Autodesk Inventor part; units mm, degrees
(part 2 of 3)
sketch "Sketch1" plane through (0, 0, 0) normal (0, 1, 0) x (-1, 0, 0)
  circle A0 centre (0, 0) radius 7.7717
  line L0 (3.8714, 3.1643) -> (5.8376, 5.1305)
  line L1 (3.1643, 3.8714) -> (5.1305, 5.8376)
  line L2 (-3.1643, -3.8714) -> (-5.1305, -5.8376)
  line L3 (-3.8714, -3.1643) -> (-5.8376, -5.1305)
  line L4 (3.1643, -3.8714) -> (5.1305, -5.8376)
  line L5 (5.8376, -5.1305) -> (3.8714, -3.1643)
  line L6 (-3.8714, 3.1643) -> (-5.8376, 5.1305)
  line L7 (-3.1643, 3.8714) -> (-5.1305, 5.8376)
  line L8 (0, 0) -> (0, -3.4995) construction
  line L9 (0, 0) -> (1.6685, -1.6685) construction
  circle A1 centre (0, 0) radius 5
  line L10 (0, 0) -> (2.6888, 2.6888) construction
  line L11 (4.7918, 7.3512) -> (4.9104, 7.3218)
  line L12 (4.9104, 7.3218) -> (4.97, 7.3308)
  line L13 (4.97, 7.3308) -> (5.0192, 7.3467)
  line L14 (5.0192, 7.3467) -> (5.0629, 7.3663)
  line L15 (5.0629, 7.3663) -> (5.1027, 7.3884)
  line L16 (5.1027, 7.3884) -> (5.1747, 7.4379)
  line L17 (5.1747, 7.4379) -> (5.2391, 7.4925)
  line L18 (5.2391, 7.4925) -> (5.2982, 7.5509)
  line L19 (5.2982, 7.5509) -> (5.3528, 7.6123)
  line L20 (5.3528, 7.6123) -> (5.456, 7.7394)
  line L21 (5.456, 7.7394) -> (5.5742, 7.8558)
  line L22 (5.5742, 7.8558) -> (5.7038, 7.964)
  line L23 (5.7038, 7.964) -> (5.8421, 8.0657)
  line L24 (5.8421, 8.0657) -> (5.9879, 8.1615)
  line L25 (5.9879, 8.1615) -> (6.1405, 8.2518)
  line L26 (6.1405, 8.2518) -> (6.2994, 8.3368)
  line L27 (6.2994, 8.3368) -> (6.4641, 8.4166)
  line L28 (6.4641, 8.4166) -> (6.6342, 8.4914)
  line L29 (6.6342, 8.4914) -> (6.8096, 8.5612)
  line L30 (6.8096, 8.5612) -> (6.9898, 8.6259)
  line L31 (6.9898, 8.6259) -> (7.1281, 8.6711)
  line L32 (7.1281, 8.6711) -> (7.4493, 8.3968)
  line L33 (7.4493, 8.3968) -> (7.4262, 8.2531)
  line L34 (7.4262, 8.2531) -> (7.3905, 8.065)
  line L35 (7.3905, 8.065) -> (7.3491, 7.8809)
  line L36 (7.3491, 7.8809) -> (7.3018, 7.7011)
  line L37 (7.3018, 7.7011) -> (7.2487, 7.526)
  line L38 (7.2487, 7.526) -> (7.1896, 7.3558)
  line L39 (7.1896, 7.3558) -> (7.1243, 7.1909)
  line L40 (7.1243, 7.1909) -> (7.0525, 7.0319)
  line L41 (7.0525, 7.0319) -> (6.9737, 6.8794)
  line L42 (6.9737, 6.8794) -> (6.8871, 6.7345)
  line L43 (6.8871, 6.7345) -> (6.7906, 6.5995)
  line L44 (6.7906, 6.5995) -> (6.6812, 6.4777)
  line L45 (6.6812, 6.4777) -> (6.6291, 6.4142)
  line L46 (6.6291, 6.4142) -> (6.5807, 6.3467)
  line L47 (6.5807, 6.3467) -> (6.5369, 6.2745)
  line L48 (6.5369, 6.2745) -> (6.4992, 6.1957)
  line L49 (6.4992, 6.1957) -> (6.4836, 6.1529)
  line L50 (6.4836, 6.1529) -> (6.4711, 6.1067)
  line L51 (6.4711, 6.1067) -> (6.4631, 6.0556)
  line L52 (6.4631, 6.0556) -> (6.4635, 5.9953)
  line L53 (6.4635, 5.9953) -> (6.5111, 5.8828)
  line L54 (6.5111, 5.8828) -> (6.829, 5.5107)
  line L55 (6.829, 5.5107) -> (6.9326, 5.446)
  line L56 (6.9326, 5.446) -> (6.9921, 5.4362)
  line L57 (6.9921, 5.4362) -> (7.0439, 5.4361)
  line L58 (7.0439, 5.4361) -> (7.0914, 5.4413)
  line L59 (7.0914, 5.4413) -> (7.1361, 5.45)
  line L60 (7.1361, 5.45) -> (7.2198, 5.4748)
  line L61 (7.2198, 5.4748) -> (7.298, 5.5068)
  line L62 (7.298, 5.5068) -> (7.3722, 5.5441)
  line L63 (7.3722, 5.5441) -> (7.4432, 5.5856)
  line L64 (7.4432, 5.5856) -> (7.5805, 5.6746)
  line L65 (7.5805, 5.6746) -> (7.729, 5.7488)
  line L66 (7.729, 5.7488) -> (7.8856, 5.8117)
  line L67 (7.8856, 5.8117) -> (8.0486, 5.8656)
  line L68 (8.0486, 5.8656) -> (8.2169, 5.9116)
  line L69 (8.2169, 5.9116) -> (8.3899, 5.9504)
  line L70 (8.3899, 5.9504) -> (8.5673, 5.9821)
  line L71 (8.5673, 5.9821) -> (8.7486, 6.0072)
  line L72 (8.7486, 6.0072) -> (8.9335, 6.0257)
  line L73 (8.9335, 6.0257) -> (9.1218, 6.0379)
  line L74 (9.1218, 6.0379) -> (9.3133, 6.0437)
  line L75 (9.3133, 6.0437) -> (9.4588, 6.044)
  line L76 (9.4588, 6.044) -> (9.6794, 5.6839)
  line L77 (9.6794, 5.6839) -> (9.6131, 5.5544)
  line L78 (9.6131, 5.5544) -> (9.521, 5.3864)
  line L79 (9.521, 5.3864) -> (9.4247, 5.2242)
  line L80 (9.4247, 5.2242) -> (9.3242, 5.0678)
  line L81 (9.3242, 5.0678) -> (9.2196, 4.9177)
  line L82 (9.2196, 4.9177) -> (9.1108, 4.7741)
  line L83 (9.1108, 4.7741) -> (8.9977, 4.6375)
  line L84 (8.9977, 4.6375) -> (8.8803, 4.5084)
  line L85 (8.8803, 4.5084) -> (8.7582, 4.3877)
  line L86 (8.7582, 4.3877) -> (8.6311, 4.2767)
  line L87 (8.6311, 4.2767) -> (8.4976, 4.1781)
  line L88 (8.4976, 4.1781) -> (8.3559, 4.0961)
  line L89 (8.3559, 4.0961) -> (8.2867, 4.0517)
  line L90 (8.2867, 4.0517) -> (8.2199, 4.0026)
  line L91 (8.2199, 4.0026) -> (8.1559, 3.9474)
  line L92 (8.1559, 3.9474) -> (8.0957, 3.8841)
  line L93 (8.0957, 3.8841) -> (8.0676, 3.8482)
  line L94 (8.0676, 3.8482) -> (8.0414, 3.8082)
  line L95 (8.0414, 3.8082) -> (8.0181, 3.762)
  line L96 (8.0181, 3.762) -> (7.9998, 3.7046)
  line L97 (7.9998, 3.7046) -> (8.0103, 3.5829)
  line L98 (8.0103, 3.5829) -> (8.1976, 3.1307)
  line L99 (8.1976, 3.1307) -> (8.2762, 3.0372)
  line L100 (8.2762, 3.0372) -> (8.3298, 3.0095)
  line L101 (8.3298, 3.0095) -> (8.3789, 2.9934)
  line L102 (8.3789, 2.9934) -> (8.4258, 2.9836)
  line L103 (8.4258, 2.9836) -> (8.471, 2.9781)
  line L104 (8.471, 2.9781) -> (8.5583, 2.9758)
  line L105 (8.5583, 2.9758) -> (8.6426, 2.9821)
  line L106 (8.6426, 2.9821) -> (8.7246, 2.9946)
  line L107 (8.7246, 2.9946) -> (8.8049, 3.0122)
  line L108 (8.8049, 3.0122) -> (8.9631, 3.0544)
  line L109 (8.9631, 3.0544) -> (9.1272, 3.0791)
  line L110 (9.1272, 3.0791) -> (9.2956, 3.0905)
  line L111 (9.2956, 3.0905) -> (9.4672, 3.0914)
  line L112 (9.4672, 3.0914) -> (9.6415, 3.0832)
  line L113 (9.6415, 3.0832) -> (9.8181, 3.0665)
  line L114 (9.8181, 3.0665) -> (9.9966, 3.0419)
  line L115 (9.9966, 3.0419) -> (10.1767, 3.0097)
  line L116 (10.1767, 3.0097) -> (10.3583, 2.9702)
  line L117 (10.3583, 2.9702) -> (10.5412, 2.9236)
  line L118 (10.5412, 2.9236) -> (10.7251, 2.87)
  line L119 (10.7251, 2.87) -> (10.8635, 2.8253)
  line L120 (10.8635, 2.8253) -> (10.9621, 2.4146)
  line L121 (10.9621, 2.4146) -> (10.859, 2.3119)
  line L122 (10.859, 2.3119) -> (10.7195, 2.1807)
  line L123 (10.7195, 2.1807) -> (10.5778, 2.0561)
  line L124 (10.5778, 2.0561) -> (10.4339, 1.9385)
  line L125 (10.4339, 1.9385) -> (10.288, 1.828)
  line L126 (10.288, 1.828) -> (10.1401, 1.725)
  line L127 (10.1401, 1.725) -> (9.9904, 1.63)
  line L128 (9.9904, 1.63) -> (9.8388, 1.5436)
  line L129 (9.8388, 1.5436) -> (9.6855, 1.4665)
  line L130 (9.6855, 1.4665) -> (9.5302, 1.4002)
  line L131 (9.5302, 1.4002) -> (9.3728, 1.3477)
  line L132 (9.3728, 1.3477) -> (9.2127, 1.3135)
  line L133 (9.2127, 1.3135) -> (9.1332, 1.2927)
  line L134 (9.1332, 1.2927) -> (9.0544, 1.2666)
  line L135 (9.0544, 1.2666) -> (8.9765, 1.2339)
  line L136 (8.9765, 1.2339) -> (8.8997, 1.1923)
  line L137 (8.8997, 1.1923) -> (8.8619, 1.1668)
  line L138 (8.8619, 1.1668) -> (8.8247, 1.1368)
  line L139 (8.8247, 1.1368) -> (8.7882, 1.1002)
  line L140 (8.7882, 1.1002) -> (8.753, 1.0512)
  line L141 (8.753, 1.0512) -> (8.7254, 0.9322)
  line L142 (8.7254, 0.9322) -> (8.7638, 0.4443)
  line L143 (8.7638, 0.4443) -> (8.8097, 0.331)
  line L144 (8.8097, 0.331) -> (8.8521, 0.2881)
  line L145 (8.8521, 0.2881) -> (8.8939, 0.2576)
  line L146 (8.8939, 0.2576) -> (8.9354, 0.2339)
  line L147 (8.9354, 0.2339) -> (8.9767, 0.2146)
  line L148 (8.9767, 0.2146) -> (9.059, 0.1855)
  line L149 (9.059, 0.1855) -> (9.1411, 0.1654)
  line L150 (9.1411, 0.1654) -> (9.223, 0.152)
  line L151 (9.223, 0.152) -> (9.3048, 0.1439)
  line L152 (9.3048, 0.1439) -> (9.4682, 0.1351)
  line L153 (9.4682, 0.1351) -> (9.6319, 0.1079)
  line L154 (9.6319, 0.1079) -> (9.7956, 0.0667)
  line L155 (9.7956, 0.0667) -> (9.9592, 0.0146)
  line L156 (9.9592, 0.0146) -> (10.1224, -0.0471)
  line L157 (10.1224, -0.0471) -> (10.2851, -0.1175)
  line L158 (10.2851, -0.1175) -> (10.4473, -0.1961)
  line L159 (10.4473, -0.1961) -> (10.6087, -0.2824)
  line L160 (10.6087, -0.2824) -> (10.7692, -0.3761)
  line L161 (10.7692, -0.3761) -> (10.9287, -0.4769)
  line L162 (10.9287, -0.4769) -> (11.087, -0.5847)
  line L163 (11.087, -0.5847) -> (11.2049, -0.67)
  line L164 (11.2049, -0.67) -> (11.1718, -1.0911)
  line L165 (11.1718, -1.0911) -> (11.042, -1.1569)
  line L166 (11.042, -1.1569) -> (10.8687, -1.2386)
  line L167 (10.8687, -1.2386) -> (10.6955, -1.3132)
  line L168 (10.6955, -1.3132) -> (10.5223, -1.3807)
  line L169 (10.5223, -1.3807) -> (10.3493, -1.4406)
  line L170 (10.3493, -1.4406) -> (10.1769, -1.4929)
  line L171 (10.1769, -1.4929) -> (10.0051, -1.5369)
  line L172 (10.0051, -1.5369) -> (9.8343, -1.5723)
  line L173 (9.8343, -1.5723) -> (9.6646, -1.5983)
  line L174 (9.6646, -1.5983) -> (9.4965, -1.6134)
  line L175 (9.4965, -1.6134) -> (9.3305, -1.6146)
  line L176 (9.3305, -1.6146) -> (9.1677, -1.5977)
  line L177 (9.1677, -1.5977) -> (9.0856, -1.5929)
  line L178 (9.0856, -1.5929) -> (9.0026, -1.5934)
  line L179 (9.0026, -1.5934) -> (8.9185, -1.6004)
  line L180 (8.9185, -1.6004) -> (8.8326, -1.6162)
  line L181 (8.8326, -1.6162) -> (8.7888, -1.6288)
  line L182 (8.7888, -1.6288) -> (8.744, -1.6458)
  line L183 (8.744, -1.6458) -> (8.698, -1.6694)
  line L184 (8.698, -1.6694) -> (8.6495, -1.7051)
  line L185 (8.6495, -1.7051) -> (8.5864, -1.8098)
  line L186 (8.5864, -1.8098) -> (8.4722, -2.2857)
  line L187 (8.4722, -2.2857) -> (8.4808, -2.4075)
  line L188 (8.4808, -2.4075) -> (8.5079, -2.4614)
  line L189 (8.5079, -2.4614) -> (8.5382, -2.5033)
  line L190 (8.5382, -2.5033) -> (8.5703, -2.5388)
  line L191 (8.5703, -2.5388) -> (8.6037, -2.5698)
  line L192 (8.6037, -2.5698) -> (8.673, -2.6229)
  line L193 (8.673, -2.6229) -> (8.7448, -2.6674)
  line L194 (8.7448, -2.6674) -> (8.8185, -2.7055)
  line L195 (8.8185, -2.7055) -> (8.8938, -2.7385)
  line L196 (8.8938, -2.7385) -> (9.0466, -2.7973)
  line L197 (9.0466, -2.7973) -> (9.1938, -2.8738)
  line L198 (9.1938, -2.8738) -> (9.3368, -2.9636)
  line L199 (9.3368, -2.9636) -> (9.4762, -3.0637)
  line L200 (9.4762, -3.0637) -> (9.6124, -3.1728)
  line L201 (9.6124, -3.1728) -> (9.7454, -3.2901)
  line L202 (9.7454, -3.2901) -> (9.8754, -3.4149)
  line L203 (9.8754, -3.4149) -> (10.0022, -3.5468)
  line L204 (10.0022, -3.5468) -> (10.1259, -3.6855)
  line L205 (10.1259, -3.6855) -> (10.2464, -3.8307)
  line L206 (10.2464, -3.8307) -> (10.3637, -3.9822)
  line L207 (10.3637, -3.9822) -> (10.4494, -4.0997)
  line L208 (10.4494, -4.0997) -> (10.2878, -4.4899)
  line L209 (10.2878, -4.4899) -> (10.1441, -4.5124)
  line L210 (10.1441, -4.5124) -> (9.954, -4.5366)
  line L211 (9.954, -4.5366) -> (9.7662, -4.554)
  line L212 (9.7662, -4.554) -> (9.5806, -4.5647)
  line L213 (9.5806, -4.5647) -> (9.3976, -4.5683)
  line L214 (9.3976, -4.5683) -> (9.2175, -4.5646)
  line L215 (9.2175, -4.5646) -> (9.0405, -4.5535)
  line L216 (9.0405, -4.5535) -> (8.8671, -4.5343)
  line L217 (8.8671, -4.5343) -> (8.6977, -4.5066)
  line L218 (8.6977, -4.5066) -> (8.5331, -4.469)
  line L219 (8.5331, -4.469) -> (8.3749, -4.4189)
  line L220 (8.3749, -4.4189) -> (8.2253, -4.3525)
  line L221 (8.2253, -4.3525) -> (8.1487, -4.3226)
  line L222 (8.1487, -4.3226) -> (8.0696, -4.2974)
  line L223 (8.0696, -4.2974) -> (7.9874, -4.278)
  line L224 (7.9874, -4.278) -> (7.9008, -4.2666)
  line L225 (7.9008, -4.2666) -> (7.8553, -4.2649)
  line L226 (7.8553, -4.2649) -> (7.8075, -4.2673)
  line L227 (7.8075, -4.2673) -> (7.7564, -4.2755)
  line L228 (7.7564, -4.2755) -> (7.6992, -4.2945)
  line L229 (7.6992, -4.2945) -> (7.607, -4.3745)
  line L230 (7.607, -4.3745) -> (7.3512, -4.7918)
  line L231 (7.3512, -4.7918) -> (7.3218, -4.9104)
  line L232 (7.3218, -4.9104) -> (7.3308, -4.97)
  line L233 (7.3308, -4.97) -> (7.3467, -5.0192)
  line L234 (7.3467, -5.0192) -> (7.3663, -5.0629)
  line L235 (7.3663, -5.0629) -> (7.3884, -5.1027)
  line L236 (7.3884, -5.1027) -> (7.4379, -5.1747)
  line L237 (7.4379, -5.1747) -> (7.4925, -5.2391)
  line L238 (7.4925, -5.2391) -> (7.5509, -5.2982)
  line L239 (7.5509, -5.2982) -> (7.6123, -5.3528)
  line L240 (7.6123, -5.3528) -> (7.7394, -5.456)
  line L241 (7.7394, -5.456) -> (7.8558, -5.5742)
  line L242 (7.8558, -5.5742) -> (7.964, -5.7037)
  line L243 (7.964, -5.7037) -> (8.0657, -5.8421)
  line L244 (8.0657, -5.8421) -> (8.1615, -5.9879)
  line L245 (8.1615, -5.9879) -> (8.2518, -6.1405)
  line L246 (8.2518, -6.1405) -> (8.3368, -6.2994)
  line L247 (8.3368, -6.2994) -> (8.4166, -6.4641)
  line L248 (8.4166, -6.4641) -> (8.4914, -6.6342)
  line L249 (8.4914, -6.6342) -> (8.5612, -6.8096)
  line L250 (8.5612, -6.8096) -> (8.6259, -6.9898)
  line L251 (8.6259, -6.9898) -> (8.6711, -7.1281)
  line L252 (8.6711, -7.1281) -> (8.3968, -7.4493)
  line L253 (8.3968, -7.4493) -> (8.2532, -7.4262)
  line L254 (8.2532, -7.4262) -> (8.065, -7.3905)
  line L255 (8.065, -7.3905) -> (7.8809, -7.3491)
  line L256 (7.8809, -7.3491) -> (7.7011, -7.3018)
  line L257 (7.7011, -7.3018) -> (7.526, -7.2487)
  line L258 (7.526, -7.2487) -> (7.3558, -7.1896)
  line L259 (7.3558, -7.1896) -> (7.1909, -7.1243)
  line L260 (7.1909, -7.1243) -> (7.0319, -7.0525)
  line L261 (7.0319, -7.0525) -> (6.8794, -6.9737)
  line L262 (6.8794, -6.9737) -> (6.7345, -6.8871)
  line L263 (6.7345, -6.8871) -> (6.5995, -6.7906)
  line L264 (6.5995, -6.7906) -> (6.4777, -6.6812)
  line L265 (6.4777, -6.6812) -> (6.4142, -6.6291)
  line L266 (6.4142, -6.6291) -> (6.3467, -6.5807)
  line L267 (6.3467, -6.5807) -> (6.2745, -6.5369)
  line L268 (6.2745, -6.5369) -> (6.1957, -6.4992)
  line L269 (6.1957, -6.4992) -> (6.1529, -6.4836)
  line L270 (6.1529, -6.4836) -> (6.1067, -6.4711)
  line L271 (6.1067, -6.4711) -> (6.0556, -6.4631)
  line L272 (6.0556, -6.4631) -> (5.9953, -6.4635)
  line L273 (5.9953, -6.4635) -> (5.8828, -6.5111)
  line L274 (5.8828, -6.5111) -> (5.5107, -6.829)
  line L275 (5.5107, -6.829) -> (5.446, -6.9326)
  line L276 (5.446, -6.9326) -> (5.4362, -6.9921)
  line L277 (5.4362, -6.9921) -> (5.4361, -7.0438)
  line L278 (5.4361, -7.0438) -> (5.4413, -7.0914)
  line L279 (5.4413, -7.0914) -> (5.45, -7.1361)
  line L280 (5.45, -7.1361) -> (5.4748, -7.2198)
  line L281 (5.4748, -7.2198) -> (5.5068, -7.298)
  line L282 (5.5068, -7.298) -> (5.5441, -7.3722)
  line L283 (5.5441, -7.3722) -> (5.5856, -7.4432)
  line L284 (5.5856, -7.4432) -> (5.6746, -7.5805)
  line L285 (5.6746, -7.5805) -> (5.7488, -7.729)
  line L286 (5.7488, -7.729) -> (5.8117, -7.8856)
  line L287 (5.8117, -7.8856) -> (5.8656, -8.0486)
  line L288 (5.8656, -8.0486) -> (5.9117, -8.2169)
  line L289 (5.9117, -8.2169) -> (5.9504, -8.3899)
  line L290 (5.9504, -8.3899) -> (5.9821, -8.5673)
  line L291 (5.9821, -8.5673) -> (6.0072, -8.7486)
  line L292 (6.0072, -8.7486) -> (6.0257, -8.9335)
  line L293 (6.0257, -8.9335) -> (6.0379, -9.1218)
  line L294 (6.0379, -9.1218) -> (6.0437, -9.3133)
  line L295 (6.0437, -9.3133) -> (6.044, -9.4588)
  line L296 (6.044, -9.4588) -> (5.6839, -9.6794)
  line L297 (5.6839, -9.6794) -> (5.5544, -9.6131)
  line L298 (5.5544, -9.6131) -> (5.3865, -9.521)
  line L299 (5.3865, -9.521) -> (5.2242, -9.4247)
  line L300 (5.2242, -9.4247) -> (5.0678, -9.3242)
  line L301 (5.0678, -9.3242) -> (4.9177, -9.2196)
  line L302 (4.9177, -9.2196) -> (4.7741, -9.1108)
  line L303 (4.7741, -9.1108) -> (4.6375, -8.9977)
  line L304 (4.6375, -8.9977) -> (4.5084, -8.8803)
  line L305 (4.5084, -8.8803) -> (4.3877, -8.7583)
  line L306 (4.3877, -8.7583) -> (4.2766, -8.6311)
  line L307 (4.2766, -8.6311) -> (4.1781, -8.4976)
  line L308 (4.1781, -8.4976) -> (4.0961, -8.3559)
  line L309 (4.0961, -8.3559) -> (4.0517, -8.2867)
  line L310 (4.0517, -8.2867) -> (4.0026, -8.2199)
  line L311 (4.0026, -8.2199) -> (3.9474, -8.1559)
  line L312 (3.9474, -8.1559) -> (3.8841, -8.0957)
  line L313 (3.8841, -8.0957) -> (3.8482, -8.0676)
  line L314 (3.8482, -8.0676) -> (3.8082, -8.0414)
  line L315 (3.8082, -8.0414) -> (3.762, -8.0181)
  line L316 (3.762, -8.0181) -> (3.7046, -7.9998)
  line L317 (3.7046, -7.9998) -> (3.5829, -8.0103)
  line L318 (3.5829, -8.0103) -> (3.1307, -8.1976)
  line L319 (3.1307, -8.1976) -> (3.0372, -8.2762)
  line L320 (3.0372, -8.2762) -> (3.0095, -8.3298)
  line L321 (3.0095, -8.3298) -> (2.9934, -8.3789)
  line L322 (2.9934, -8.3789) -> (2.9836, -8.4258)
  line L323 (2.9836, -8.4258) -> (2.9781, -8.471)
  line L324 (2.9781, -8.471) -> (2.9758, -8.5583)
  line L325 (2.9758, -8.5583) -> (2.9821, -8.6425)
  line L326 (2.9821, -8.6425) -> (2.9946, -8.7246)
  line L327 (2.9946, -8.7246) -> (3.0122, -8.8049)
  line L328 (3.0122, -8.8049) -> (3.0544, -8.9631)
  line L329 (3.0544, -8.9631) -> (3.0791, -9.1272)
  line L330 (3.0791, -9.1272) -> (3.0905, -9.2956)
  line L331 (3.0905, -9.2956) -> (3.0914, -9.4672)
  line L332 (3.0914, -9.4672) -> (3.0832, -9.6415)
  line L333 (3.0832, -9.6415) -> (3.0665, -9.8181)
  line L334 (3.0665, -9.8181) -> (3.0419, -9.9966)
  line L335 (3.0419, -9.9966) -> (3.0097, -10.1767)
  line L336 (3.0097, -10.1767) -> (2.9702, -10.3583)
  line L337 (2.9702, -10.3583) -> (2.9236, -10.5412)
  line L338 (2.9236, -10.5412) -> (2.87, -10.7251)
  line L339 (2.87, -10.7251) -> (2.8253, -10.8635)
  line L340 (2.8253, -10.8635) -> (2.4146, -10.9621)
  line L341 (2.4146, -10.9621) -> (2.3119, -10.859)
  line L342 (2.3119, -10.859) -> (2.1807, -10.7195)
  line L343 (2.1807, -10.7195) -> (2.0561, -10.5778)
  line L344 (2.0561, -10.5778) -> (1.9385, -10.4339)
  line L345 (1.9385, -10.4339) -> (1.828, -10.288)
  line L346 (1.828, -10.288) -> (1.725, -10.1401)
  line L347 (1.725, -10.1401) -> (1.63, -9.9904)
  line L348 (1.63, -9.9904) -> (1.5436, -9.8388)
  line L349 (1.5436, -9.8388) -> (1.4665, -9.6855)
  line L350 (1.4665, -9.6855) -> (1.4002, -9.5302)
  line L351 (1.4002, -9.5302) -> (1.3477, -9.3728)
  line L352 (1.3477, -9.3728) -> (1.3135, -9.2127)
  line L353 (1.3135, -9.2127) -> (1.2927, -9.1332)
  line L354 (1.2927, -9.1332) -> (1.2666, -9.0544)
  line L355 (1.2666, -9.0544) -> (1.2339, -8.9765)
  line L356 (1.2339, -8.9765) -> (1.1923, -8.8997)
  line L357 (1.1923, -8.8997) -> (1.1668, -8.8619)
  line L358 (1.1668, -8.8619) -> (1.1368, -8.8247)
  line L359 (1.1368, -8.8247) -> (1.1002, -8.7882)
  line L360 (1.1002, -8.7882) -> (1.0512, -8.753)
  line L361 (1.0512, -8.753) -> (0.9322, -8.7254)
  line L362 (0.9322, -8.7254) -> (0.4443, -8.7638)
  line L363 (0.4443, -8.7638) -> (0.331, -8.8097)
  line L364 (0.331, -8.8097) -> (0.2881, -8.8521)
  line L365 (0.2881, -8.8521) -> (0.2576, -8.8938)
  line L366 (0.2576, -8.8938) -> (0.2339, -8.9354)
  line L367 (0.2339, -8.9354) -> (0.2146, -8.9767)
  line L368 (0.2146, -8.9767) -> (0.1855, -9.059)
  line L369 (0.1855, -9.059) -> (0.1654, -9.1411)
  line L370 (0.1654, -9.1411) -> (0.152, -9.223)
  line L371 (0.152, -9.223) -> (0.1439, -9.3048)
  line L372 (0.1439, -9.3048) -> (0.1351, -9.4682)
  line L373 (0.1351, -9.4682) -> (0.1079, -9.6319)
  line L374 (0.1079, -9.6319) -> (0.0667, -9.7956)
  line L375 (0.0667, -9.7956) -> (0.0146, -9.9592)
  line L376 (0.0146, -9.9592) -> (-0.0471, -10.1224)
  line L377 (-0.0471, -10.1224) -> (-0.1175, -10.2851)
  line L378 (-0.1175, -10.2851) -> (-0.1961, -10.4473)
  line L379 (-0.1961, -10.4473) -> (-0.2824, -10.6087)
  line L380 (-0.2824, -10.6087) -> (-0.3761, -10.7692)
  line L381 (-0.3761, -10.7692) -> (-0.4769, -10.9287)
  line L382 (-0.4769, -10.9287) -> (-0.5847, -11.087)
  line L383 (-0.5847, -11.087) -> (-0.67, -11.2049)
  line L384 (-0.67, -11.2049) -> (-1.091, -11.1718)
  line L385 (-1.091, -11.1718) -> (-1.1569, -11.042)
  line L386 (-1.1569, -11.042) -> (-1.2386, -10.8687)
  line L387 (-1.2386, -10.8687) -> (-1.3132, -10.6954)
  line L388 (-1.3132, -10.6954) -> (-1.3807, -10.5223)
  line L389 (-1.3807, -10.5223) -> (-1.4406, -10.3493)
  line L390 (-1.4406, -10.3493) -> (-1.4929, -10.1769)
  line L391 (-1.4929, -10.1769) -> (-1.5369, -10.0051)
  line L392 (-1.5369, -10.0051) -> (-1.5723, -9.8343)
  line L393 (-1.5723, -9.8343) -> (-1.5983, -9.6646)
  line L394 (-1.5983, -9.6646) -> (-1.6133, -9.4965)
  line L395 (-1.6133, -9.4965) -> (-1.6146, -9.3305)
  line L396 (-1.6146, -9.3305) -> (-1.5977, -9.1677)
  line L397 (-1.5977, -9.1677) -> (-1.5929, -9.0856)
  line L398 (-1.5929, -9.0856) -> (-1.5934, -9.0026)
  line L399 (-1.5934, -9.0026) -> (-1.6004, -8.9185)
  line L400 (-1.6004, -8.9185) -> (-1.6162, -8.8326)
  line L401 (-1.6162, -8.8326) -> (-1.6288, -8.7888)
  line L402 (-1.6288, -8.7888) -> (-1.6458, -8.7441)
  line L403 (-1.6458, -8.7441) -> (-1.6694, -8.698)
  line L404 (-1.6694, -8.698) -> (-1.7051, -8.6495)
  line L405 (-1.7051, -8.6495) -> (-1.8098, -8.5864)
  line L406 (-1.8098, -8.5864) -> (-2.2857, -8.4722)
  line L407 (-2.2857, -8.4722) -> (-2.4075, -8.4808)
  line L408 (-2.4075, -8.4808) -> (-2.4614, -8.5079)
  line L409 (-2.4614, -8.5079) -> (-2.5033, -8.5382)
  line L410 (-2.5033, -8.5382) -> (-2.5388, -8.5703)
  line L411 (-2.5388, -8.5703) -> (-2.5698, -8.6036)
  line L412 (-2.5698, -8.6036) -> (-2.6229, -8.673)
  line L413 (-2.6229, -8.673) -> (-2.6674, -8.7448)
  line L414 (-2.6674, -8.7448) -> (-2.7055, -8.8185)
  line L415 (-2.7055, -8.8185) -> (-2.7385, -8.8938)
  line L416 (-2.7385, -8.8938) -> (-2.7973, -9.0466)
  line L417 (-2.7973, -9.0466) -> (-2.8738, -9.1938)
  line L418 (-2.8738, -9.1938) -> (-2.9636, -9.3368)
  line L419 (-2.9636, -9.3368) -> (-3.0637, -9.4762)
  line L420 (-3.0637, -9.4762) -> (-3.1728, -9.6124)
  line L421 (-3.1728, -9.6124) -> (-3.2901, -9.7454)
  line L422 (-3.2901, -9.7454) -> (-3.4149, -9.8754)
  line L423 (-3.4149, -9.8754) -> (-3.5468, -10.0022)
  line L424 (-3.5468, -10.0022) -> (-3.6855, -10.1259)
  line L425 (-3.6855, -10.1259) -> (-3.8307, -10.2464)
  line L426 (-3.8307, -10.2464) -> (-3.9822, -10.3637)
  line L427 (-3.9822, -10.3637) -> (-4.0997, -10.4494)
  line L428 (-4.0997, -10.4494) -> (-4.4899, -10.2878)
  line L429 (-4.4899, -10.2878) -> (-4.5124, -10.1441)
  line L430 (-4.5124, -10.1441) -> (-4.5366, -9.954)
  line L431 (-4.5366, -9.954) -> (-4.5541, -9.7662)
  line L432 (-4.5541, -9.7662) -> (-4.5647, -9.5806)
  line L433 (-4.5647, -9.5806) -> (-4.5683, -9.3976)
  line L434 (-4.5683, -9.3976) -> (-4.5646, -9.2175)
  line L435 (-4.5646, -9.2175) -> (-4.5535, -9.0405)
  line L436 (-4.5535, -9.0405) -> (-4.5343, -8.8671)
  line L437 (-4.5343, -8.8671) -> (-4.5066, -8.6977)
  line L438 (-4.5066, -8.6977) -> (-4.469, -8.5331)
  line L439 (-4.469, -8.5331) -> (-4.4189, -8.3749)
  line L440 (-4.4189, -8.3749) -> (-4.3525, -8.2253)
  line L441 (-4.3525, -8.2253) -> (-4.3226, -8.1487)
  line L442 (-4.3226, -8.1487) -> (-4.2974, -8.0696)
  line L443 (-4.2974, -8.0696) -> (-4.278, -7.9874)
  line L444 (-4.278, -7.9874) -> (-4.2666, -7.9008)
  line L445 (-4.2666, -7.9008) -> (-4.2649, -7.8553)
  line L446 (-4.2649, -7.8553) -> (-4.2673, -7.8075)
  line L447 (-4.2673, -7.8075) -> (-4.2755, -7.7564)
  line L448 (-4.2755, -7.7564) -> (-4.2945, -7.6992)
  line L449 (-4.2945, -7.6992) -> (-4.3745, -7.6069)
  line L450 (-4.3745, -7.6069) -> (-4.7918, -7.3512)
  line L451 (-4.7918, -7.3512) -> (-4.9104, -7.3218)
  line L452 (-4.9104, -7.3218) -> (-4.97, -7.3308)
  line L453 (-4.97, -7.3308) -> (-5.0192, -7.3467)
  line L454 (-5.0192, -7.3467) -> (-5.0629, -7.3663)
  line L455 (-5.0629, -7.3663) -> (-5.1027, -7.3884)
  line L456 (-5.1027, -7.3884) -> (-5.1747, -7.4379)
  line L457 (-5.1747, -7.4379) -> (-5.2391, -7.4925)
  line L458 (-5.2391, -7.4925) -> (-5.2982, -7.5509)
  line L459 (-5.2982, -7.5509) -> (-5.3528, -7.6123)
  line L460 (-5.3528, -7.6123) -> (-5.456, -7.7394)
  line L461 (-5.456, -7.7394) -> (-5.5742, -7.8558)
  line L462 (-5.5742, -7.8558) -> (-5.7037, -7.964)
  line L463 (-5.7037, -7.964) -> (-5.8421, -8.0657)
  line L464 (-5.8421, -8.0657) -> (-5.9879, -8.1615)
  line L465 (-5.9879, -8.1615) -> (-6.1405, -8.2518)
  line L466 (-6.1405, -8.2518) -> (-6.2994, -8.3368)
  line L467 (-6.2994, -8.3368) -> (-6.4641, -8.4166)
  line L468 (-6.4641, -8.4166) -> (-6.6342, -8.4914)
  line L469 (-6.6342, -8.4914) -> (-6.8096, -8.5612)
  line L470 (-6.8096, -8.5612) -> (-6.9898, -8.6259)
  line L471 (-6.9898, -8.6259) -> (-7.1281, -8.6711)
  line L472 (-7.1281, -8.6711) -> (-7.4493, -8.3968)
  line L473 (-7.4493, -8.3968) -> (-7.4262, -8.2532)
  line L474 (-7.4262, -8.2532) -> (-7.3905, -8.065)
  line L475 (-7.3905, -8.065) -> (-7.3491, -7.8809)
  line L476 (-7.3491, -7.8809) -> (-7.3018, -7.7011)
  line L477 (-7.3018, -7.7011) -> (-7.2487, -7.526)
  line L478 (-7.2487, -7.526) -> (-7.1896, -7.3558)
  line L479 (-7.1896, -7.3558) -> (-7.1243, -7.1909)
  line L480 (-7.1243, -7.1909) -> (-7.0525, -7.0319)
  line L481 (-7.0525, -7.0319) -> (-6.9737, -6.8794)
  line L482 (-6.9737, -6.8794) -> (-6.8871, -6.7345)
  line L483 (-6.8871, -6.7345) -> (-6.7906, -6.5995)
  line L484 (-6.7906, -6.5995) -> (-6.6812, -6.4777)
  line L485 (-6.6812, -6.4777) -> (-6.6291, -6.4142)
  line L486 (-6.6291, -6.4142) -> (-6.5807, -6.3467)
  line L487 (-6.5807, -6.3467) -> (-6.5369, -6.2745)
  line L488 (-6.5369, -6.2745) -> (-6.4992, -6.1957)
  line L489 (-6.4992, -6.1957) -> (-6.4836, -6.1529)
  line L490 (-6.4836, -6.1529) -> (-6.4711, -6.1067)
  line L491 (-6.4711, -6.1067) -> (-6.4631, -6.0556)
  line L492 (-6.4631, -6.0556) -> (-6.4635, -5.9953)
  line L493 (-6.4635, -5.9953) -> (-6.5111, -5.8828)
  line L494 (-6.5111, -5.8828) -> (-6.829, -5.5107)
  line L495 (-6.829, -5.5107) -> (-6.9326, -5.446)
  line L496 (-6.9326, -5.446) -> (-6.9921, -5.4362)
  line L497 (-6.9921, -5.4362) -> (-7.0438, -5.4361)
  line L498 (-7.0438, -5.4361) -> (-7.0914, -5.4413)
  line L499 (-7.0914, -5.4413) -> (-7.1361, -5.45)
  line L500 (-7.1361, -5.45) -> (-7.2198, -5.4749)
  line L501 (-7.2198, -5.4749) -> (-7.298, -5.5068)
  line L502 (-7.298, -5.5068) -> (-7.3722, -5.5441)
  line L503 (-7.3722, -5.5441) -> (-7.4432, -5.5856)
  line L504 (-7.4432, -5.5856) -> (-7.5805, -5.6746)
  line L505 (-7.5805, -5.6746) -> (-7.729, -5.7488)
  line L506 (-7.729, -5.7488) -> (-7.8856, -5.8117)
  line L507 (-7.8856, -5.8117) -> (-8.0486, -5.8656)
  line L508 (-8.0486, -5.8656) -> (-8.2169, -5.9117)
  line L509 (-8.2169, -5.9117) -> (-8.3899, -5.9504)
  line L510 (-8.3899, -5.9504) -> (-8.5673, -5.9821)
  line L511 (-8.5673, -5.9821) -> (-8.7486, -6.0072)
  line L512 (-8.7486, -6.0072) -> (-8.9335, -6.0257)
  line L513 (-8.9335, -6.0257) -> (-9.1218, -6.0379)
  line L514 (-9.1218, -6.0379) -> (-9.3133, -6.0437)
  line L515 (-9.3133, -6.0437) -> (-9.4588, -6.044)
  line L516 (-9.4588, -6.044) -> (-9.6794, -5.6839)
  line L517 (-9.6794, -5.6839) -> (-9.6131, -5.5544)
  line L518 (-9.6131, -5.5544) -> (-9.521, -5.3865)
  line L519 (-9.521, -5.3865) -> (-9.4247, -5.2242)
  line L520 (-9.4247, -5.2242) -> (-9.3242, -5.0678)
  line L521 (-9.3242, -5.0678) -> (-9.2196, -4.9177)
  line L522 (-9.2196, -4.9177) -> (-9.1108, -4.7741)
  line L523 (-9.1108, -4.7741) -> (-8.9977, -4.6375)
  line L524 (-8.9977, -4.6375) -> (-8.8803, -4.5084)
  line L525 (-8.8803, -4.5084) -> (-8.7583, -4.3877)
  line L526 (-8.7583, -4.3877) -> (-8.6311, -4.2767)
  line L527 (-8.6311, -4.2767) -> (-8.4976, -4.1781)
  line L528 (-8.4976, -4.1781) -> (-8.3559, -4.0961)
  line L529 (-8.3559, -4.0961) -> (-8.2867, -4.0517)
  line L530 (-8.2867, -4.0517) -> (-8.2199, -4.0026)
  line L531 (-8.2199, -4.0026) -> (-8.1559, -3.9474)
  line L532 (-8.1559, -3.9474) -> (-8.0957, -3.8841)
  line L533 (-8.0957, -3.8841) -> (-8.0676, -3.8482)
  line L534 (-8.0676, -3.8482) -> (-8.0414, -3.8082)
  line L535 (-8.0414, -3.8082) -> (-8.0181, -3.762)
  line L536 (-8.0181, -3.762) -> (-7.9998, -3.7046)
  line L537 (-7.9998, -3.7046) -> (-8.0103, -3.5829)
  line L538 (-8.0103, -3.5829) -> (-8.1976, -3.1307)
  line L539 (-8.1976, -3.1307) -> (-8.2762, -3.0372)
  line L540 (-8.2762, -3.0372) -> (-8.3298, -3.0095)
  line L541 (-8.3298, -3.0095) -> (-8.3789, -2.9934)
  line L542 (-8.3789, -2.9934) -> (-8.4258, -2.9836)
  line L543 (-8.4258, -2.9836) -> (-8.471, -2.9781)
  line L544 (-8.471, -2.9781) -> (-8.5583, -2.9758)
  line L545 (-8.5583, -2.9758) -> (-8.6426, -2.9821)
  line L546 (-8.6426, -2.9821) -> (-8.7246, -2.9946)
  line L547 (-8.7246, -2.9946) -> (-8.8049, -3.0122)
  line L548 (-8.8049, -3.0122) -> (-8.9631, -3.0544)
  line L549 (-8.9631, -3.0544) -> (-9.1272, -3.0791)
  line L550 (-9.1272, -3.0791) -> (-9.2956, -3.0905)
  line L551 (-9.2956, -3.0905) -> (-9.4672, -3.0914)
  line L552 (-9.4672, -3.0914) -> (-9.6415, -3.0832)
  line L553 (-9.6415, -3.0832) -> (-9.8181, -3.0665)
  line L554 (-9.8181, -3.0665) -> (-9.9966, -3.0419)
  line L555 (-9.9966, -3.0419) -> (-10.1767, -3.0097)
  line L556 (-10.1767, -3.0097) -> (-10.3583, -2.9702)
  line L557 (-10.3583, -2.9702) -> (-10.5412, -2.9236)
  line L558 (-10.5412, -2.9236) -> (-10.7251, -2.87)
  line L559 (-10.7251, -2.87) -> (-10.8635, -2.8253)
  line L560 (-10.8635, -2.8253) -> (-10.9621, -2.4146)
  line L561 (-10.9621, -2.4146) -> (-10.859, -2.3119)
  line L562 (-10.859, -2.3119) -> (-10.7195, -2.1807)
  line L563 (-10.7195, -2.1807) -> (-10.5778, -2.0561)
  line L564 (-10.5778, -2.0561) -> (-10.4339, -1.9385)
  line L565 (-10.4339, -1.9385) -> (-10.288, -1.828)
  line L566 (-10.288, -1.828) -> (-10.1401, -1.725)
  line L567 (-10.1401, -1.725) -> (-9.9904, -1.63)
  line L568 (-9.9904, -1.63) -> (-9.8388, -1.5436)
  line L569 (-9.8388, -1.5436) -> (-9.6855, -1.4665)
  line L570 (-9.6855, -1.4665) -> (-9.5302, -1.4002)
  line L571 (-9.5302, -1.4002) -> (-9.3728, -1.3477)
  line L572 (-9.3728, -1.3477) -> (-9.2127, -1.3135)
  line L573 (-9.2127, -1.3135) -> (-9.1332, -1.2927)
  line L574 (-9.1332, -1.2927) -> (-9.0544, -1.2666)
  line L575 (-9.0544, -1.2666) -> (-8.9765, -1.2339)
  line L576 (-8.9765, -1.2339) -> (-8.8997, -1.1923)
  line L577 (-8.8997, -1.1923) -> (-8.8619, -1.1668)
  line L578 (-8.8619, -1.1668) -> (-8.8247, -1.1368)
  line L579 (-8.8247, -1.1368) -> (-8.7882, -1.1002)
  line L580 (-8.7882, -1.1002) -> (-8.753, -1.0512)
  line L581 (-8.753, -1.0512) -> (-8.7254, -0.9322)
  line L582 (-8.7254, -0.9322) -> (-8.7638, -0.4443)
  line L583 (-8.7638, -0.4443) -> (-8.8097, -0.331)
  line L584 (-8.8097, -0.331) -> (-8.8521, -0.2882)
  line L585 (-8.8521, -0.2882) -> (-8.8939, -0.2576)
  line L586 (-8.8939, -0.2576) -> (-8.9354, -0.2339)
  line L587 (-8.9354, -0.2339) -> (-8.9767, -0.2146)
  line L588 (-8.9767, -0.2146) -> (-9.059, -0.1855)
  line L589 (-9.059, -0.1855) -> (-9.1411, -0.1654)
  line L590 (-9.1411, -0.1654) -> (-9.223, -0.152)
  line L591 (-9.223, -0.152) -> (-9.3048, -0.1439)
  line L592 (-9.3048, -0.1439) -> (-9.4682, -0.1351)
  line L593 (-9.4682, -0.1351) -> (-9.6319, -0.1079)
  line L594 (-9.6319, -0.1079) -> (-9.7956, -0.0667)
  line L595 (-9.7956, -0.0667) -> (-9.9592, -0.0146)
  line L596 (-9.9592, -0.0146) -> (-10.1224, 0.0471)
  line L597 (-10.1224, 0.0471) -> (-10.2851, 0.1175)
  line L598 (-10.2851, 0.1175) -> (-10.4473, 0.1961)
  line L599 (-10.4473, 0.1961) -> (-10.6087, 0.2824)
  line L600 (-10.6087, 0.2824) -> (-10.7692, 0.3761)
  line L601 (-10.7692, 0.3761) -> (-10.9287, 0.4769)
  line L602 (-10.9287, 0.4769) -> (-11.087, 0.5847)
  line L603 (-11.087, 0.5847) -> (-11.2049, 0.67)
  line L604 (-11.2049, 0.67) -> (-11.1718, 1.091)
  line L605 (-11.1718, 1.091) -> (-11.042, 1.1569)
  line L606 (-11.042, 1.1569) -> (-10.8688, 1.2386)
  line L607 (-10.8688, 1.2386) -> (-10.6955, 1.3133)
  line L608 (-10.6955, 1.3133) -> (-10.5223, 1.3807)
  line L609 (-10.5223, 1.3807) -> (-10.3493, 1.4406)
  line L610 (-10.3493, 1.4406) -> (-10.1769, 1.4929)
  line L611 (-10.1769, 1.4929) -> (-10.0051, 1.5369)
  line L612 (-10.0051, 1.5369) -> (-9.8343, 1.5723)
  line L613 (-9.8343, 1.5723) -> (-9.6646, 1.5983)
  line L614 (-9.6646, 1.5983) -> (-9.4965, 1.6133)
  line L615 (-9.4965, 1.6133) -> (-9.3305, 1.6146)
  line L616 (-9.3305, 1.6146) -> (-9.1677, 1.5977)
  line L617 (-9.1677, 1.5977) -> (-9.0856, 1.5929)
  line L618 (-9.0856, 1.5929) -> (-9.0026, 1.5934)
  line L619 (-9.0026, 1.5934) -> (-8.9185, 1.6004)
  line L620 (-8.9185, 1.6004) -> (-8.8326, 1.6162)
  line L621 (-8.8326, 1.6162) -> (-8.7888, 1.6288)
  line L622 (-8.7888, 1.6288) -> (-8.7441, 1.6458)
  line L623 (-8.7441, 1.6458) -> (-8.698, 1.6694)
  line L624 (-8.698, 1.6694) -> (-8.6495, 1.7051)
  line L625 (-8.6495, 1.7051) -> (-8.5864, 1.8098)
  line L626 (-8.5864, 1.8098) -> (-8.4722, 2.2857)
  line L627 (-8.4722, 2.2857) -> (-8.4808, 2.4075)
  line L628 (-8.4808, 2.4075) -> (-8.5079, 2.4614)
  line L629 (-8.5079, 2.4614) -> (-8.5382, 2.5033)
  line L630 (-8.5382, 2.5033) -> (-8.5703, 2.5388)
  line L631 (-8.5703, 2.5388) -> (-8.6037, 2.5698)
  line L632 (-8.6037, 2.5698) -> (-8.673, 2.6229)
  line L633 (-8.673, 2.6229) -> (-8.7448, 2.6674)
  line L634 (-8.7448, 2.6674) -> (-8.8185, 2.7055)
  line L635 (-8.8185, 2.7055) -> (-8.8938, 2.7385)
  line L636 (-8.8938, 2.7385) -> (-9.0466, 2.7973)
  line L637 (-9.0466, 2.7973) -> (-9.1939, 2.8738)
  line L638 (-9.1939, 2.8738) -> (-9.3368, 2.9636)
  line L639 (-9.3368, 2.9636) -> (-9.4762, 3.0637)
  line L640 (-9.4762, 3.0637) -> (-9.6124, 3.1728)
  line L641 (-9.6124, 3.1728) -> (-9.7454, 3.2901)
  line L642 (-9.7454, 3.2901) -> (-9.8754, 3.4149)
  line L643 (-9.8754, 3.4149) -> (-10.0022, 3.5468)
  line L644 (-10.0022, 3.5468) -> (-10.1259, 3.6855)
  line L645 (-10.1259, 3.6855) -> (-10.2464, 3.8307)
  line L646 (-10.2464, 3.8307) -> (-10.3637, 3.9822)
  line L647 (-10.3637, 3.9822) -> (-10.4494, 4.0997)
  line L648 (-10.4494, 4.0997) -> (-10.2878, 4.4899)
  line L649 (-10.2878, 4.4899) -> (-10.144, 4.5124)
  line L650 (-10.144, 4.5124) -> (-9.9541, 4.5366)
  line L651 (-9.9541, 4.5366) -> (-9.7662, 4.554)
  line L652 (-9.7662, 4.554) -> (-9.5806, 4.5647)
  line L653 (-9.5806, 4.5647) -> (-9.3976, 4.5682)
  line L654 (-9.3976, 4.5682) -> (-9.2175, 4.5646)
  line L655 (-9.2175, 4.5646) -> (-9.0405, 4.5535)
  line L656 (-9.0405, 4.5535) -> (-8.8671, 4.5343)
  line L657 (-8.8671, 4.5343) -> (-8.6977, 4.5066)
  line L658 (-8.6977, 4.5066) -> (-8.5331, 4.469)
  line L659 (-8.5331, 4.469) -> (-8.3749, 4.4189)
  line L660 (-8.3749, 4.4189) -> (-8.2253, 4.3525)
  line L661 (-8.2253, 4.3525) -> (-8.1487, 4.3226)
  line L662 (-8.1487, 4.3226) -> (-8.0696, 4.2974)
  line L663 (-8.0696, 4.2974) -> (-7.9874, 4.278)
  line L664 (-7.9874, 4.278) -> (-7.9008, 4.2666)
  line L665 (-7.9008, 4.2666) -> (-7.8553, 4.2649)
  line L666 (-7.8553, 4.2649) -> (-7.8075, 4.2673)
  line L667 (-7.8075, 4.2673) -> (-7.7564, 4.2755)
  line L668 (-7.7564, 4.2755) -> (-7.6992, 4.2945)
  line L669 (-7.6992, 4.2945) -> (-7.6069, 4.3745)
  line L670 (-7.6069, 4.3745) -> (-7.3512, 4.7918)
  line L671 (-7.3512, 4.7918) -> (-7.3218, 4.9104)
  line L672 (-7.3218, 4.9104) -> (-7.3308, 4.97)
  line L673 (-7.3308, 4.97) -> (-7.3467, 5.0192)
  line L674 (-7.3467, 5.0192) -> (-7.3663, 5.0629)
  line L675 (-7.3663, 5.0629) -> (-7.3884, 5.1027)
  line L676 (-7.3884, 5.1027) -> (-7.4379, 5.1746)
  line L677 (-7.4379, 5.1746) -> (-7.4925, 5.2391)
  line L678 (-7.4925, 5.2391) -> (-7.5509, 5.2982)
  line L679 (-7.5509, 5.2982) -> (-7.6123, 5.3528)
  line L680 (-7.6123, 5.3528) -> (-7.7394, 5.456)
  line L681 (-7.7394, 5.456) -> (-7.8558, 5.5742)
  line L682 (-7.8558, 5.5742) -> (-7.964, 5.7037)
  line L683 (-7.964, 5.7037) -> (-8.0657, 5.8421)
  line L684 (-8.0657, 5.8421) -> (-8.1615, 5.9879)
  line L685 (-8.1615, 5.9879) -> (-8.2518, 6.1405)
  line L686 (-8.2518, 6.1405) -> (-8.3368, 6.2994)
  line L687 (-8.3368, 6.2994) -> (-8.4166, 6.4641)
  line L688 (-8.4166, 6.4641) -> (-8.4914, 6.6342)
  line L689 (-8.4914, 6.6342) -> (-8.5612, 6.8096)
  line L690 (-8.5612, 6.8096) -> (-8.6259, 6.9898)
  line L691 (-8.6259, 6.9898) -> (-8.6711, 7.1281)
  line L692 (-8.6711, 7.1281) -> (-8.3968, 7.4493)
  line L693 (-8.3968, 7.4493) -> (-8.2532, 7.4262)
  line L694 (-8.2532, 7.4262) -> (-8.065, 7.3905)
  line L695 (-8.065, 7.3905) -> (-7.8809, 7.3491)
  line L696 (-7.8809, 7.3491) -> (-7.7011, 7.3018)
  line L697 (-7.7011, 7.3018) -> (-7.526, 7.2487)
  line L698 (-7.526, 7.2487) -> (-7.3558, 7.1896)
  line L699 (-7.3558, 7.1896) -> (-7.1909, 7.1243)
  line L700 (-7.1909, 7.1243) -> (-7.0319, 7.0525)
  line L701 (-7.0319, 7.0525) -> (-6.8794, 6.9737)
  line L702 (-6.8794, 6.9737) -> (-6.7345, 6.8871)
  line L703 (-6.7345, 6.8871) -> (-6.5995, 6.7906)
  line L704 (-6.5995, 6.7906) -> (-6.4777, 6.6812)
  line L705 (-6.4777, 6.6812) -> (-6.4142, 6.6291)
  line L706 (-6.4142, 6.6291) -> (-6.3467, 6.5807)
  line L707 (-6.3467, 6.5807) -> (-6.2745, 6.5369)
  line L708 (-6.2745, 6.5369) -> (-6.1957, 6.4992)
  line L709 (-6.1957, 6.4992) -> (-6.1529, 6.4836)
  line L710 (-6.1529, 6.4836) -> (-6.1067, 6.4711)
  line L711 (-6.1067, 6.4711) -> (-6.0556, 6.4631)
  line L712 (-6.0556, 6.4631) -> (-5.9953, 6.4635)
  line L713 (-5.9953, 6.4635) -> (-5.8828, 6.5111)
  line L714 (-5.8828, 6.5111) -> (-5.5107, 6.829)
  line L715 (-5.5107, 6.829) -> (-5.446, 6.9326)
  line L716 (-5.446, 6.9326) -> (-5.4362, 6.9921)
  line L717 (-5.4362, 6.9921) -> (-5.4361, 7.0438)
  line L718 (-5.4361, 7.0438) -> (-5.4413, 7.0914)
  line L719 (-5.4413, 7.0914) -> (-5.45, 7.1361)
  line L720 (-5.45, 7.1361) -> (-5.4748, 7.2198)
  line L721 (-5.4748, 7.2198) -> (-5.5068, 7.298)
  line L722 (-5.5068, 7.298) -> (-5.5441, 7.3722)
  line L723 (-5.5441, 7.3722) -> (-5.5856, 7.4432)
  line L724 (-5.5856, 7.4432) -> (-5.6746, 7.5805)
  line L725 (-5.6746, 7.5805) -> (-5.7488, 7.729)
  line L726 (-5.7488, 7.729) -> (-5.8117, 7.8856)
  line L727 (-5.8117, 7.8856) -> (-5.8656, 8.0486)
  line L728 (-5.8656, 8.0486) -> (-5.9117, 8.2169)
  line L729 (-5.9117, 8.2169) -> (-5.9504, 8.3899)
  line L730 (-5.9504, 8.3899) -> (-5.9821, 8.5673)
  line L731 (-5.9821, 8.5673) -> (-6.0072, 8.7486)
  line L732 (-6.0072, 8.7486) -> (-6.0257, 8.9335)
  line L733 (-6.0257, 8.9335) -> (-6.0379, 9.1218)
  line L734 (-6.0379, 9.1218) -> (-6.0437, 9.3133)
  line L735 (-6.0437, 9.3133) -> (-6.044, 9.4588)
  line L736 (-6.044, 9.4588) -> (-5.6839, 9.6794)
  line L737 (-5.6839, 9.6794) -> (-5.5544, 9.6131)
  line L738 (-5.5544, 9.6131) -> (-5.3865, 9.521)
  line L739 (-5.3865, 9.521) -> (-5.2242, 9.4247)
  line L740 (-5.2242, 9.4247) -> (-5.0678, 9.3242)
  line L741 (-5.0678, 9.3242) -> (-4.9177, 9.2196)
  line L742 (-4.9177, 9.2196) -> (-4.7741, 9.1108)
  line L743 (-4.7741, 9.1108) -> (-4.6375, 8.9977)
  line L744 (-4.6375, 8.9977) -> (-4.5084, 8.8803)
  line L745 (-4.5084, 8.8803) -> (-4.3877, 8.7583)
  line L746 (-4.3877, 8.7583) -> (-4.2767, 8.6311)
  line L747 (-4.2767, 8.6311) -> (-4.1781, 8.4976)
  line L748 (-4.1781, 8.4976) -> (-4.0961, 8.3559)
  line L749 (-4.0961, 8.3559) -> (-4.0517, 8.2867)
  line L750 (-4.0517, 8.2867) -> (-4.0026, 8.2199)
  line L751 (-4.0026, 8.2199) -> (-3.9474, 8.1559)
  line L752 (-3.9474, 8.1559) -> (-3.8841, 8.0957)
  line L753 (-3.8841, 8.0957) -> (-3.8482, 8.0676)
  line L754 (-3.8482, 8.0676) -> (-3.8082, 8.0414)
  line L755 (-3.8082, 8.0414) -> (-3.762, 8.0181)
  line L756 (-3.762, 8.0181) -> (-3.7046, 7.9998)
  line L757 (-3.7046, 7.9998) -> (-3.5829, 8.0103)
  line L758 (-3.5829, 8.0103) -> (-3.1307, 8.1976)
  line L759 (-3.1307, 8.1976) -> (-3.0372, 8.2762)
  line L760 (-3.0372, 8.2762) -> (-3.0095, 8.3298)
  line L761 (-3.0095, 8.3298) -> (-2.9934, 8.3789)
  line L762 (-2.9934, 8.3789) -> (-2.9836, 8.4258)
  line L763 (-2.9836, 8.4258) -> (-2.9781, 8.471)
  line L764 (-2.9781, 8.471) -> (-2.9758, 8.5583)
  line L765 (-2.9758, 8.5583) -> (-2.9821, 8.6426)
  line L766 (-2.9821, 8.6426) -> (-2.9946, 8.7246)
  line L767 (-2.9946, 8.7246) -> (-3.0122, 8.8049)
  line L768 (-3.0122, 8.8049) -> (-3.0544, 8.9631)
  line L769 (-3.0544, 8.9631) -> (-3.0791, 9.1272)
  line L770 (-3.0791, 9.1272) -> (-3.0905, 9.2956)
  line L771 (-3.0905, 9.2956) -> (-3.0914, 9.4672)
  line L772 (-3.0914, 9.4672) -> (-3.0832, 9.6415)
  line L773 (-3.0832, 9.6415) -> (-3.0665, 9.8181)
  line L774 (-3.0665, 9.8181) -> (-3.0419, 9.9966)
  line L775 (-3.0419, 9.9966) -> (-3.0097, 10.1767)
  line L776 (-3.0097, 10.1767) -> (-2.9702, 10.3583)
  line L777 (-2.9702, 10.3583) -> (-2.9236, 10.5412)
  line L778 (-2.9236, 10.5412) -> (-2.87, 10.7251)
  line L779 (-2.87, 10.7251) -> (-2.8253, 10.8635)
  line L780 (-2.8253, 10.8635) -> (-2.4146, 10.9621)
  line L781 (-2.4146, 10.9621) -> (-2.3119, 10.859)
  line L782 (-2.3119, 10.859) -> (-2.1807, 10.7195)
  line L783 (-2.1807, 10.7195) -> (-2.0561, 10.5778)
  line L784 (-2.0561, 10.5778) -> (-1.9385, 10.4339)
  line L785 (-1.9385, 10.4339) -> (-1.828, 10.288)
  line L786 (-1.828, 10.288) -> (-1.725, 10.1401)
  line L787 (-1.725, 10.1401) -> (-1.63, 9.9904)
  line L788 (-1.63, 9.9904) -> (-1.5436, 9.8388)
  line L789 (-1.5436, 9.8388) -> (-1.4665, 9.6855)
  line L790 (-1.4665, 9.6855) -> (-1.4002, 9.5302)
  line L791 (-1.4002, 9.5302) -> (-1.3477, 9.3728)
  line L792 (-1.3477, 9.3728) -> (-1.3135, 9.2127)
  line L793 (-1.3135, 9.2127) -> (-1.2927, 9.1332)
  line L794 (-1.2927, 9.1332) -> (-1.2666, 9.0544)
  line L795 (-1.2666, 9.0544) -> (-1.2339, 8.9765)
  line L796 (-1.2339, 8.9765) -> (-1.1923, 8.8997)
  line L797 (-1.1923, 8.8997) -> (-1.1668, 8.8619)
  line L798 (-1.1668, 8.8619) -> (-1.1368, 8.8247)
  line L799 (-1.1368, 8.8247) -> (-1.1002, 8.7882)
  line L800 (-1.1002, 8.7882) -> (-1.0512, 8.753)
  line L801 (-1.0512, 8.753) -> (-0.9322, 8.7254)
  line L802 (-0.9322, 8.7254) -> (-0.4443, 8.7638)
  line L803 (-0.4443, 8.7638) -> (-0.3311, 8.8097)
  line L804 (-0.3311, 8.8097) -> (-0.2881, 8.8521)
  line L805 (-0.2881, 8.8521) -> (-0.2576, 8.8939)
  line L806 (-0.2576, 8.8939) -> (-0.2339, 8.9354)
  line L807 (-0.2339, 8.9354) -> (-0.2146, 8.9767)
  line L808 (-0.2146, 8.9767) -> (-0.1855, 9.059)
  line L809 (-0.1855, 9.059) -> (-0.1654, 9.1411)
  line L810 (-0.1654, 9.1411) -> (-0.152, 9.223)
  line L811 (-0.152, 9.223) -> (-0.1439, 9.3048)
  line L812 (-0.1439, 9.3048) -> (-0.1351, 9.4682)
  line L813 (-0.1351, 9.4682) -> (-0.1079, 9.6319)
  line L814 (-0.1079, 9.6319) -> (-0.0667, 9.7956)
  line L815 (-0.0667, 9.7956) -> (-0.0146, 9.9592)
  line L816 (-0.0146, 9.9592) -> (0.0471, 10.1224)
  line L817 (0.0471, 10.1224) -> (0.1175, 10.2851)
  line L818 (0.1175, 10.2851) -> (0.1961, 10.4473)
  line L819 (0.1961, 10.4473) -> (0.2824, 10.6087)
  line L820 (0.2824, 10.6087) -> (0.3761, 10.7692)
  line L821 (0.3761, 10.7692) -> (0.4769, 10.9287)
  line L822 (0.4769, 10.9287) -> (0.5847, 11.087)
  line L823 (0.5847, 11.087) -> (0.67, 11.2049)
  line L824 (0.67, 11.2049) -> (1.0911, 11.1718)
  line L825 (1.0911, 11.1718) -> (1.1569, 11.042)
  line L826 (1.1569, 11.042) -> (1.2386, 10.8688)
  line L827 (1.2386, 10.8688) -> (1.3132, 10.6955)
  line L828 (1.3132, 10.6955) -> (1.3807, 10.5223)
  line L829 (1.3807, 10.5223) -> (1.4406, 10.3493)
  line L830 (1.4406, 10.3493) -> (1.4929, 10.1769)
  line L831 (1.4929, 10.1769) -> (1.5369, 10.0051)
  line L832 (1.5369, 10.0051) -> (1.5723, 9.8343)
  line L833 (1.5723, 9.8343) -> (1.5983, 9.6646)
  line L834 (1.5983, 9.6646) -> (1.6133, 9.4965)
  line L835 (1.6133, 9.4965) -> (1.6146, 9.3305)
  line L836 (1.6146, 9.3305) -> (1.5977, 9.1677)
  line L837 (1.5977, 9.1677) -> (1.5929, 9.0857)
  line L838 (1.5929, 9.0857) -> (1.5934, 9.0027)
  line L839 (1.5934, 9.0027) -> (1.6004, 8.9184)
  line L840 (1.6004, 8.9184) -> (1.6162, 8.8326)
  line L841 (1.6162, 8.8326) -> (1.6288, 8.7888)
  line L842 (1.6288, 8.7888) -> (1.6458, 8.7441)
  line L843 (1.6458, 8.7441) -> (1.6694, 8.698)
  line L844 (1.6694, 8.698) -> (1.7051, 8.6495)
  line L845 (1.7051, 8.6495) -> (1.8098, 8.5864)
  line L846 (1.8098, 8.5864) -> (2.2857, 8.4722)
  line L847 (2.2857, 8.4722) -> (2.4075, 8.4808)
  line L848 (2.4075, 8.4808) -> (2.4614, 8.5079)
  line L849 (2.4614, 8.5079) -> (2.5033, 8.5382)
  line L850 (2.5033, 8.5382) -> (2.5388, 8.5703)
  line L851 (2.5388, 8.5703) -> (2.5698, 8.6037)
  line L852 (2.5698, 8.6037) -> (2.6229, 8.673)
  line L853 (2.6229, 8.673) -> (2.6674, 8.7448)
  line L854 (2.6674, 8.7448) -> (2.7055, 8.8185)
  line L855 (2.7055, 8.8185) -> (2.7385, 8.8938)
  line L856 (2.7385, 8.8938) -> (2.7973, 9.0466)
  line L857 (2.7973, 9.0466) -> (2.8738, 9.1938)
  line L858 (2.8738, 9.1938) -> (2.9636, 9.3368)
  line L859 (2.9636, 9.3368) -> (3.0637, 9.4762)
  line L860 (3.0637, 9.4762) -> (3.1728, 9.6124)
  line L861 (3.1728, 9.6124) -> (3.2901, 9.7454)
  line L862 (3.2901, 9.7454) -> (3.4149, 9.8754)
  line L863 (3.4149, 9.8754) -> (3.5468, 10.0022)
  line L864 (3.5468, 10.0022) -> (3.6855, 10.1259)
  line L865 (3.6855, 10.1259) -> (3.8307, 10.2464)
  line L866 (3.8307, 10.2464) -> (3.9822, 10.3637)
  line L867 (3.9822, 10.3637) -> (4.0997, 10.4494)
  line L868 (4.0997, 10.4494) -> (4.4899, 10.2878)
  line L869 (4.4899, 10.2878) -> (4.5124, 10.1441)
  line L870 (4.5124, 10.1441) -> (4.5366, 9.954)
  line L871 (4.5366, 9.954) -> (4.554, 9.7662)
  line L872 (4.554, 9.7662) -> (4.5647, 9.5806)
  line L873 (4.5647, 9.5806) -> (4.5683, 9.3976)
  line L874 (4.5683, 9.3976) -> (4.5646, 9.2175)
  line L875 (4.5646, 9.2175) -> (4.5535, 9.0405)
  line L876 (4.5535, 9.0405) -> (4.5343, 8.8671)
  line L877 (4.5343, 8.8671) -> (4.5066, 8.6977)
  line L878 (4.5066, 8.6977) -> (4.4689, 8.5331)
  line L879 (4.4689, 8.5331) -> (4.4189, 8.3749)
  line L880 (4.4189, 8.3749) -> (4.3525, 8.2253)
  line L881 (4.3525, 8.2253) -> (4.3226, 8.1487)
  line L882 (4.3226, 8.1487) -> (4.2974, 8.0697)
  line L883 (4.2974, 8.0697) -> (4.278, 7.9874)
  line L884 (4.278, 7.9874) -> (4.2666, 7.9008)
  line L885 (4.2666, 7.9008) -> (4.2649, 7.8553)
  line L886 (4.2649, 7.8553) -> (4.2673, 7.8075)
  line L887 (4.2673, 7.8075) -> (4.2755, 7.7564)
  line L888 (4.2755, 7.7564) -> (4.2945, 7.6992)
  line L889 (4.2945, 7.6992) -> (4.3745, 7.6069)
  line L890 (4.3745, 7.6069) -> (4.7918, 7.3512)
  circle A2 centre (0, 0) radius 0.5
  line L891 (-0.8805, -11.1883) -> (0.8805, 11.1883) construction
  line L892 (11.1883, -0.8805) -> (-11.1883, 0.8805) construction
  point P0 (0, 0)
  point P1 (0, 0)
  point P2 (0, 0)
  point P3 (0, 0)
  dimension "d7" = 1
  dimension "d17" = 10
  dimension "d6" = 1
  dimension "d8" = 1
  dimension "d16" = 4.5
  dimension "d18" = 45
  constraints: 22 end point, 7 coincident, 4 collinear, 1 parallel, 1 perpendicular, 1 vertical, 27 other
  measures "d6" distance between parallel lines of L0 L1
  measures "d8" distance between parallel lines of L5 L4
  measures "d18" angle of L8 L9